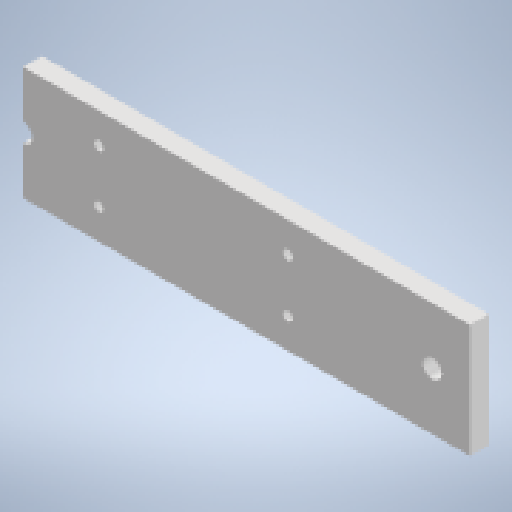
# Autodesk Inventor part: arm counterweight
Saved by Autodesk Inventor 2023 (Build 270158000, 158)
## iProperties
Created: 2023-10-16
Part Number: arm counterweight
Material: Generic
Document SubType Name: Modeling
Designer: Nate
Density: 1 g/cm^3
Appearance: Default
Author: Nate
Autodesk Inventor part; units mm, degrees
ref_plane "YZ Plane" through (0, 0, 0) normal (1, 0, 0) x (0, 1, 0)
ref_plane "XZ Plane" through (0, 0, 0) normal (0, 1, 0) x (-1, 0, 0)
ref_plane "XY Plane" through (0, 0, 0) normal (0, 0, 1) x (1, 0, 0)
sketch "Sketch2" plane through (0, 0, 0) normal (0, 0, 1) x (1, 0, 0)
  line L0 (0, 0) -> (150.0124, 0)
  line L1 (150.0124, 0) -> (150.0124, 38.1)
  line L2 (150.0124, 38.1) -> (0, 38.1)
  line L3 (0, 38.1) -> (0, 0)
  circle A0 centre (137.3124, 19.05) radius 3.175
  circle A1 centre (25.4, 27.94) radius 1.5875
  circle A2 centre (88.9, 27.94) radius 1.5875
  circle A3 centre (88.9, 10.16) radius 1.5875
  circle A4 centre (25.4, 10.16) radius 1.5875
  circle A5 centre (0, 19.05) radius 3.175
  point P0 (0, 22.225)
  point P1 (0, 15.875)
  dimension "d0" = 150.0124
  dimension "d1" = 38.1
  dimension "d2" = 6.35
  dimension "d3" = 3.175
  dimension "d4" = 3.175
  dimension "d5" = 3.175
  dimension "d6" = 3.175
  dimension "d7" = 6.35
  dimension "d8" = 25.4
  dimension "d9" = 10.16
  dimension "d10" = 10.16
  dimension "d12" = 88.9
  dimension "d13" = 88.9
  dimension "d14" = 10.16
  dimension "d15" = 10.16
  dimension "d16" = 25.4
  dimension "d17" = 19.05
  dimension "d18" = 12.7
  constraints: 8 end point, 6 centre point, 2 parallel, 1 horizontal, 1 midpoint, 1 perpendicular
  measures "d0" distance of L2.end L1.end
  measures "d1" distance of L1.end L0.end
  measures "d2" diameter of A0
  measures "d3" diameter of A1
  measures "d4" diameter of A2
  measures "d5" diameter of A3
  measures "d6" diameter of A4
  measures "d7" diameter of A5
  measures "d8" distance from line of A1.centre L3
  measures "d9" distance from line of L2 A1.centre
  measures "d10" distance from line of L2 A2.centre
  measures "d12" distance from line of A2.centre L3
  measures "d13" distance from line of L3 A3.centre
  measures "d14" distance from line of L0 A3.centre
  measures "d15" distance from line of L0 A4.centre
  measures "d16" distance from line of L3 A4.centre
  measures "d17" distance from line of L0 A0.centre
  measures "d18" distance from line of L1 A0.centre
extrude "Extrusion1" add sketch "Sketch2" along normal blind 6.35 contours L3 A5 L2 L1 L0
body "Solid1"
